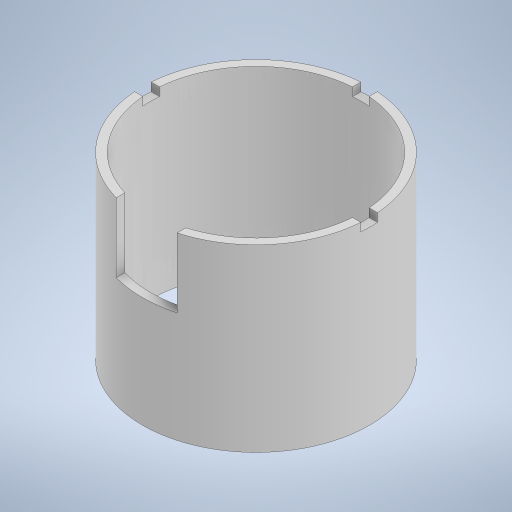
# Autodesk Inventor part: case
Saved by Autodesk Inventor 2024 (Build 280153000, 153)
## iProperties
Created: 2024-05-21
Part Number: case
Material: Generic
Document SubType Name: Modeling
Designer: ryana
Density: 1 g/cm^3
Appearance: Default
Author: ryana
Autodesk Inventor part; units mm, degrees
ref_plane "YZ Plane" through (0, 0, 0) normal (1, 0, 0) x (0, 1, 0)
ref_plane "XZ Plane" through (0, 0, 0) normal (0, 1, 0) x (-1, 0, 0)
ref_plane "XY Plane" through (0, 0, 0) normal (0, 0, 1) x (1, 0, 0)
sketch "Sketch1" plane through (0, 0, 0) normal (0, 1, 0) x (-1, 0, 0)
  circle A0 centre (0, 0) radius 41
  circle A1 centre (0, 0) radius 38
  dimension "d0" = 82
  dimension "d1" = 76
  constraints: 2 centre point, 2 coincident
  measures "d0" diameter of A0
  measures "d1" diameter of A1
extrude "Extrusion1" add sketch "Sketch1" along normal blind 65
sketch "Sketch2" plane through (0, 65, 0) normal (0, 1, 0) x (1, 0, 0)
  line L0 (41, 3) -> (41, -3)
  line L1 (41, -3) -> (-41, -3)
  line L2 (-41, -3) -> (-41, 3)
  line L3 (-41, 3) -> (41, 3)
  line L4 (41, 3) -> (-41, -3) construction
  line L5 (41, -3) -> (-41, 3) construction
  point P0 (0, 0)
  dimension "d4" = 6
  dimension "d5" = 82
  constraints: 12 end point, 2 midpoint, 2 parallel, 1 perpendicular, 1 vertical
  measures "d4" distance of L0.start L0.end
  measures "d5" distance of L0.end L1.end
extrude "Extrusion2" cut sketch "Sketch2" against normal blind 3
sketch "Sketch3" plane through (0, 65, 0) normal (0, 1, 0) x (1, 0, 0)
  line L0 (0, 0) -> (3, 0)
  line L1 (3, 0) -> (-3, 0)
  line L2 (-3, 0) -> (-3, 82)
  line L3 (-3, 82) -> (3, 82)
  line L4 (3, 82) -> (3, 0)
  dimension "d8" = 3
  dimension "d9" = 6
  dimension "d10" = 82
  constraints: 10 end point, 2 horizontal, 2 parallel, 1 perpendicular
  measures "d8" distance of L0.start L0.end
  measures "d9" distance of L2.end L3.end
  measures "d10" distance of L1.end L2.end
extrude "Extrusion3" cut sketch "Sketch3" against normal blind 3
sketch "Sketch4" plane through (0, 0, 0) normal (0, 0, 1) x (1, 0, 0)
  circle A0 centre (0, 0) radius 3
  dimension "d13" = 6
  constraints: 1 centre point, 1 coincident
  measures "d13" diameter of A0
extrude "Extrusion4" cut sketch "Sketch4" against normal blind 82
sketch "Sketch5" plane through (0, 65, 0) normal (0, 1, 0) x (1, 0, 0)
  line L0 (0, 0) -> (11, 0)
  line L1 (0, 0) -> (11, 0) construction
  line L2 (11, 0) -> (-11, 0)
  line L3 (-11, 0) -> (-11, -82)
  line L4 (-11, -82) -> (11, -82)
  line L5 (11, -82) -> (11, 0)
  dimension "d16" = 11
  dimension "d17" = 0
  dimension "d18" = 22
  dimension "d19" = 82
  constraints: 12 end point, 3 horizontal, 2 parallel, 1 collinear, 1 perpendicular
  measures "d16" distance of L0.start L0.end
  measures "d17" distance between parallel lines of L0 L1
  measures "d18" distance of L4.end L3.end
  measures "d19" distance of L3.end L2.end
extrude "Extrusion5" cut sketch "Sketch5" against normal blind 25
body "Solid1"
